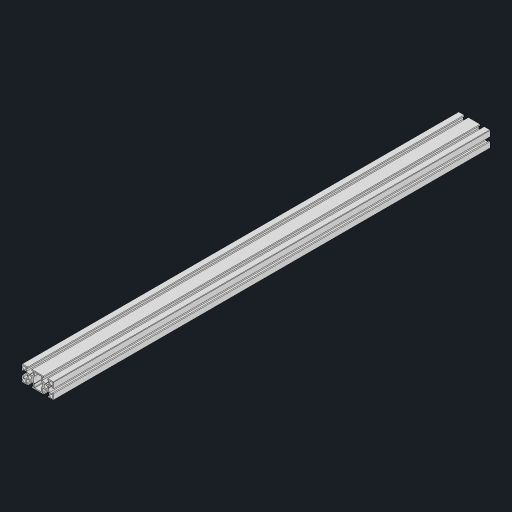
# Autodesk Inventor part: 550mm 20x40 profile
Saved by Autodesk Inventor 2024.1 (Build 281209000, 209)
## iProperties
Created: 2024-01-11
Part Number: 550mm 20x40 profile
Material: 일반
Document SubType Name: Modeling
Designer: KBU
Density: 1 g/cm^3
Appearance: 기본값
Author: KBU
Autodesk Inventor part; units mm, degrees
ref_plane "YZ Plane" through (0, 0, 0) normal (1, 0, 0) x (0, 1, 0)
ref_plane "XZ Plane" through (0, 0, 0) normal (0, 1, 0) x (-1, 0, 0)
ref_plane "XY Plane" through (0, 0, 0) normal (0, 0, 1) x (1, 0, 0)
sketch "스케치1" plane through (0, 0, 0) normal (0, 0, 1) x (1, 0, 0)
  line L0 (-19.5, -10) -> (19.5, -10)
  line L1 (20, -9.5) -> (20, 9.5)
  line L2 (19.5, 10) -> (-19.5, 10)
  line L3 (-20, 9.5) -> (-20, -9.5)
  circle A0 centre (-17, 7) radius 2
  line L4 (0, -12.143) -> (0, 11.1651)
  line L5 (28.9925, 0) -> (-24.8769, 0)
  circle A1 centre (-10, 0) radius 2.1
  line L6 (-10, 12.7543) -> (-10, -12.5913)
  line L7 (10, -12.5913) -> (10, 12.7543)
  circle A2 centre (10, 0) radius 2.1
  line L8 (-12.65, -10) -> (-12.65, -8.5)
  line L9 (-12.65, -8.5) -> (-14.15, -8.5)
  line L10 (-14.15, -8.5) -> (-14.15, -4.7403)
  line L11 (-5.85, -4.7397) -> (-5.85, -8.5)
  line L12 (-5.85, -8.5) -> (-7.35, -8.5)
  line L13 (-7.35, -8.5) -> (-7.35, -10)
  arc A3 (-5.85, -4.7397) -> (-14.15, -4.7403) centre (-9.9996, -10) ccw
  line L14 (-10, -3.05) -> (-10.25, -3.3047)
  line L15 (-10, -3.05) -> (-9.7398, -3.305)
  line L16 (12.65, -10) -> (12.65, -8.5)
  line L17 (12.65, -8.5) -> (14.15, -8.5)
  line L18 (14.15, -8.5) -> (14.15, -4.7403)
  line L19 (5.85, -4.7397) -> (5.85, -8.5)
  line L20 (5.85, -8.5) -> (7.35, -8.5)
  line L21 (7.35, -8.5) -> (7.35, -10)
  arc A4 (14.15, -4.7403) -> (5.85, -4.7397) centre (9.9996, -10) ccw
  line L22 (10, -3.05) -> (10.25, -3.3047)
  line L23 (10, -3.05) -> (9.7398, -3.305)
  line L24 (-20, 2.65) -> (-18.5, 2.65)
  line L25 (-18.5, 2.65) -> (-18.5, 4.15)
  line L26 (-18.5, 4.15) -> (-14.7403, 4.15)
  line L27 (-14.7397, -4.15) -> (-18.5, -4.15)
  line L28 (-18.5, -4.15) -> (-18.5, -2.65)
  line L29 (-18.5, -2.65) -> (-20, -2.65)
  line L30 (-13.05, 0) -> (-13.305, -0.2602)
  line L31 (-13.05, 0) -> (-13.3047, 0.25)
  arc A5 (-14.7397, -4.15) -> (-14.7403, 4.15) centre (-20, -0.0004) ccw
  line L32 (-7.35, 10) -> (-7.35, 8.5)
  line L33 (-7.35, 8.5) -> (-5.85, 8.5)
  line L34 (-5.85, 8.5) -> (-5.85, 4.7403)
  line L35 (-14.15, 4.7397) -> (-14.15, 8.5)
  line L36 (-14.15, 8.5) -> (-12.65, 8.5)
  line L37 (-12.65, 8.5) -> (-12.65, 10)
  line L38 (-10, 3.05) -> (-10.2602, 3.305)
  line L39 (-10, 3.05) -> (-9.75, 3.3047)
  arc A6 (-14.15, 4.7397) -> (-5.85, 4.7403) centre (-10.0004, 10) ccw
  line L40 (14.7397, -4.15) -> (18.5, -4.15)
  line L41 (18.5, -4.15) -> (18.5, -2.65)
  line L42 (18.5, -2.65) -> (20, -2.65)
  arc A7 (14.7403, 4.15) -> (14.7397, -4.15) centre (20, -0.0004) ccw
  line L43 (20, 2.65) -> (18.5, 2.65)
  line L44 (18.5, 2.65) -> (18.5, 4.15)
  line L45 (18.5, 4.15) -> (14.7403, 4.15)
  line L46 (13.05, 0) -> (13.305, -0.2602)
  line L47 (13.05, 0) -> (13.3047, 0.25)
  line L48 (14.15, 4.7397) -> (14.15, 8.5)
  line L49 (14.15, 8.5) -> (12.65, 8.5)
  line L50 (12.65, 8.5) -> (12.65, 10)
  arc A8 (5.85, 4.7403) -> (14.15, 4.7397) centre (10.0004, 10) ccw
  line L51 (7.35, 10) -> (7.35, 8.5)
  line L52 (7.35, 8.5) -> (5.85, 8.5)
  line L53 (5.85, 8.5) -> (5.85, 4.7403)
  line L54 (10, 3.05) -> (10.2602, 3.305)
  line L55 (10, 3.05) -> (9.75, 3.3047)
  circle A9 centre (-17, -7) radius 2
  circle A10 centre (17, 7) radius 2
  circle A11 centre (17, -7) radius 2
  line L56 (-3.85, -8.5) -> (3.85, -8.5)
  line L57 (3.85, 8.5) -> (-3.85, 8.5)
  line L58 (-4.35, -8.5) -> (4.35, 8.5) construction
  line L59 (4.35, -8.5) -> (-4.35, 8.5) construction
  arc A12 (-3.85, 8.5) -> (-4.35, 8) centre (-3.85, 8) ccw
  arc A13 (4.35, 8) -> (3.85, 8.5) centre (3.85, 8) ccw
  arc A14 (3.85, -8.5) -> (4.35, -8) centre (3.85, -8) ccw
  arc A15 (-4.35, -8) -> (-3.85, -8.5) centre (-3.85, -8) ccw
  line L60 (-4.35, 8) -> (-4.35, 4.1325)
  line L61 (-4.35, -4.3275) -> (-4.35, -8)
  line L62 (4.35, -8) -> (4.35, -4.3275)
  line L63 (4.35, 4.3275) -> (4.35, 8)
  arc A16 (4.4769, -3.9946) -> (4.4769, 3.9946) centre (0, 0) ccw
  arc A17 (-4.35, 4.1325) -> (-4.4769, -3.9946) centre (0, 0) ccw
  arc A18 (-4.35, -4.3275) -> (-4.4769, -3.9946) centre (-4.85, -4.3275) ccw
  arc A19 (4.35, 4.3275) -> (4.4769, 3.9946) centre (4.85, 4.3275) ccw
  arc A20 (4.4769, -3.9946) -> (4.35, -4.3275) centre (4.85, -4.3275) ccw
  arc A21 (-19.5, 10) -> (-20, 9.5) centre (-19.5, 9.5) ccw
  arc A22 (-20, -9.5) -> (-19.5, -10) centre (-19.5, -9.5) ccw
  arc A23 (19.5, -10) -> (20, -9.5) centre (19.5, -9.5) ccw
  arc A24 (20, 9.5) -> (19.5, 10) centre (19.5, 9.5) ccw
  point P0 (20, 10)
  point P1 (20, -10)
  point P2 (-20, 10)
  point P3 (-14.15, -6.6202)
  point P4 (-12.65, -9.25)
  point P5 (-10.0001, -3.3)
  point P6 (14.15, -6.6202)
  point P7 (12.65, -9.25)
  point P8 (10.0001, -3.3)
  point P9 (-19.25, 2.65)
  point P10 (-16.6202, 4.15)
  point P11 (-13.3, 0.0001)
  point P12 (-7.35, 9.25)
  point P13 (-5.85, 6.6202)
  point P14 (-9.9999, 3.3)
  point P15 (13.3, 0.0001)
  point P16 (19.25, 2.65)
  point P17 (16.6202, 4.15)
  point P18 (22.5913, 0)
  point P19 (9.9999, 3.3)
  point P20 (7.35, 9.25)
  point P21 (5.85, 6.6202)
  point P22 (10, 12.5913)
  point P23 (-5.85, -6.6199)
  point P24 (-4.35, -4.1325)
  point P25 (4.35, -4.1325)
  point P26 (4.35, 4.1325)
  point P27 (4.35, 6.1638)
  point P28 (-4.35, 6.0662)
  dimension "d0" = 40
  dimension "d1" = 20
  dimension "d2" = 4
  dimension "d3" = 34
  dimension "d4" = 14
  dimension "d5" = 4.2
  dimension "d6" = 20
  dimension "d8" = 4.2
  dimension "d9" = 20
  dimension "d12" = 1.5
  dimension "d13" = 6.7
  dimension "d14" = 8.3
  dimension "d15" = 5.3
  dimension "d16" = 5.3
  dimension "d17" = 8.3
  dimension "d18" = 6.7
  dimension "d19" = 0.5
  dimension "d20" = 0.25
  dimension "d23" = 180
  dimension "d27" = 180
  dimension "d29" = 1.5
  dimension "d31" = 1.5
  dimension "d32" = 0.5
  dimension "d33" = 0.5
  dimension "d34" = 0.5
  dimension "d35" = 8.7
  constraints: 128 end point, 54 point on circle, 31 point on line, 26 tangent, 25 centre point, 18 symmetric about line, 8 equal radius, 7 midpoint, 7 parallel, 6 perpendicular, 6 vertical, 4 horizontal, 1 coincident, 105 other
  measures "d0" distance of point (20, 10) point (-20, 10)
  measures "d1" distance of point (20, -10) point (20, 10)
  measures "d2" diameter of A0
  measures "d3" diameter of A0.centre L4
  measures "d4" diameter of A0.centre L5
  measures "d5" diameter of A1
  measures "d6" diameter of A1.centre L4
  measures "d8" diameter of A2
  measures "d9" diameter of A2.centre L4
  measures "d12" distance of L8.start L8.end
  measures "d13" radius of A3
  measures "d14" diameter of point (-14.15, -6.62) L6
  measures "d15" diameter of point (-12.65, -9.25) L6
  measures "d16" distance between parallel lines of L8 L13
  measures "d17" distance between parallel lines of L10 L11
  measures "d18" distance from line of L0 point (-10, -3.3)
  measures "d19" diameter of L14.end L6
  measures "d20" distance of point (-10, -3.3) L14.start
  measures "d29" distance between parallel lines of L0 L56
  measures "d31" distance between parallel lines of L2 L57
  measures "d32" radius of A12
  measures "d33" radius of A18
  measures "d34" radius of A21
  measures "d35" horizontal distance of point (4.35, 6.164) point (-4.35, 6.066)
extrude "돌출1" add sketch "스케치1" along normal blind 550 contours A22 L3 L29 L28 L27 A5 L30 L5 A1 L6 L14 A3 L10 L9 L8 L0 | L13 L12 L11 A3 L15 L6 A1 L5 A17 A18 L61 A15 L56 L4 L0 | L4 L56 A14 L62 A20 A16 L5 A2 L7 L23 A4 L19 L20 L21 L0 | L3 A21 L2 L37 L36 L35 A6 L38 L6 A1 L5 L31 A5 L26 L25 L24 | A1 L6 L39 A6 L34 L33 L32 L2 L4 L57 A12 L60 A17 L5 | L16 L17 L18 A4 L22 L7 A2 L5 L46 A7 L40 L41 L42 L1 A23 L0 | L4 L2 L51 L52 L53 A8 L55 L7 A2 L5 A16 A19 L63 A13 L57 | L7 L54 A8 L48 L49 L50 L2 A24 L1 L43 L44 L45 A7 L47 L5 A2
equation "\"d8\" = d5"
